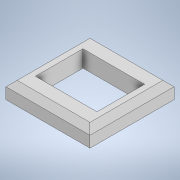
# Autodesk Inventor part: electromagnet-ending
Saved by Autodesk Inventor 2021 (Build 250183000, 183)
## iProperties
Created: 2021-01-13
Part Number: electromagnet-ending
Material: Generic
Document SubType Name: Modeling
Designer: Luke Kamols
Density: 1 g/cm^3
Appearance: Default
Author: Luke Kamols
Autodesk Inventor part; units mm, degrees
ref_plane "YZ Plane" through (0, 0, 0) normal (1, 0, 0) x (0, 1, 0)
ref_plane "XZ Plane" through (0, 0, 0) normal (0, 1, 0) x (-1, 0, 0)
ref_plane "XY Plane" through (0, 0, 0) normal (0, 0, 1) x (1, 0, 0)
sketch "Sketch1" plane through (0, 0, 0) normal (0, 1, 0) x (-1, 0, 0)
  line L0 (0, 0) -> (15, 0)
  line L1 (15, 0) -> (15, -15)
  line L2 (15, -15) -> (0, -15)
  line L3 (0, -15) -> (0, 0)
  line L4 (0, 0) -> (0, -7.5)
  line L5 (0, -7.5) -> (0.896, -7.5)
  line L6 (7.5, -11.75) -> (13, -11.75)
  line L7 (13, -11.75) -> (13, -3.25)
  line L8 (13, -3.25) -> (2, -3.25)
  line L9 (2, -3.25) -> (2, -11.75)
  line L10 (2, -11.75) -> (7.5, -11.75)
  dimension "d0" = 15
  dimension "d1" = 15
  dimension "d5" = 5.5
  dimension "d6" = 8.5
  dimension "d7" = 11
  constraints: 22 end point, 5 perpendicular, 2 parallel, 1 horizontal, 1 midpoint, 1 point on line
  measures "d0" distance of L1.end L2.end
  measures "d1" distance of L0.end L1.end
  measures "d5" distance of L6.start L6.end
  measures "d6" distance of L6.end L7.end
  measures "d7" distance of L7.end L8.end
extrude "Extrusion1" add sketch "Sketch1" along normal blind 3
chamfer "Chamfer1" distance 1 angle 45 4 edges at (0, 3, -7.5) (-7.5, 3, 0) (-15, 3, -7.5) (-7.5, 3, -15)
body "Solid1"
